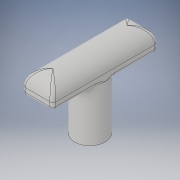
# Autodesk Inventor part: poop tray handle ver1
Saved by Autodesk Inventor 2019 (Build 230136000, 136)
## iProperties
Created: 2019-03-25
Part Number: poop tray handle ver1
Material: Generic
Document SubType Name: Modeling
Designer: aonih
Density: 1 g/cm^3
Appearance: Default
Author: aonih
Autodesk Inventor part; units mm, degrees
ref_plane "YZ Plane" through (0, 0, 0) normal (1, 0, 0) x (0, 1, 0)
ref_plane "XZ Plane" through (0, 0, 0) normal (0, 1, 0) x (-1, 0, 0)
ref_plane "XY Plane" through (0, 0, 0) normal (0, 0, 1) x (1, 0, 0)
sketch "Sketch1" plane through (0, 0, 0) normal (0, 1, 0) x (-1, 0, 0)
  circle A0 centre (0, 0) radius 5.1
  line L0 (0, 0) -> (-3.6062, -3.6062) construction
  line L1 (0, 0) -> (5.1, 0) construction
  line L2 (0, 0) -> (3.6062, 3.6062) construction
  line L3 (0, 0) -> (3.6062, -3.6062) construction
  line L4 (0, 0) -> (-3.6062, 3.6062) construction
  circle A1 centre (0, 0) radius 2.1 construction
  dimension "d7" = 135
  dimension "d8" = 5.1
  dimension "d9" = 4.2
  dimension "d10" = 3
  constraints: 10 end point, 4 point on circle, 2 centre point, 2 coincident, 1 collinear, 1 equal length, 1 horizontal, 1 perpendicular, 1 point on line
  measures "d7" angle of L0 L1
  measures "d8" distance of L0.start L0.end
  measures "d9" diameter of A1
  measures "d10" radial gap between concentric circles of A0 A1
extrude "Extrusion1" add sketch "Sketch1" along normal blind 17.5
sketch "Sketch2" plane through (0, 17.5, 0) normal (0, 1, 0) x (1, 0, 0)
  line L0 (5.1, 17.5) -> (-5.1, 17.5)
  line L1 (-5.1, 17.5) -> (-5.1, -17.5)
  line L2 (-5.1, -17.5) -> (5.1, -17.5)
  line L3 (5.1, -17.5) -> (5.1, 17.5)
  line L4 (5.1, 17.5) -> (-5.1, -17.5) construction
  line L5 (-5.1, 17.5) -> (5.1, -17.5) construction
  circle A0 centre (0, 0) radius 5.1 projected
  point P0 (-5.1, 0)
  dimension "d3" = 17.5
  dimension "d19" = 10.2
  constraints: 12 end point, 2 midpoint, 2 parallel, 1 horizontal, 1 horizontal alignment, 1 perpendicular, 1 other
  measures "d3" distance from line of point (0, 0) L2
  measures "d19" distance of L0.start L0.end
extrude "Extrusion2" add sketch "Sketch2" along normal blind 7.5
fillet "Fillet1" radius 5.1 4 edges at (5.1, 25, 0) (-5.1, 25, 0) (0, 25, 17.5) (0, 25, -17.5)
sketch "Sketch3" plane through (0, 0, 0) normal (0, -1, 0) x (1, 0, 0)
  line L0 (0, 0) -> (3.6062, -3.6062) construction
  circle A0 centre (0, 0) radius 5.1 construction
  line L1 (0, 0) -> (5.1, 0) construction
  dimension "d11" = 45
  constraints: 4 end point, 1 equal length, 1 horizontal, 2 other
  measures "d11" angle of L0 L1
hole "Hole1" at (0, 0, 0) direction (0, 1, 0) diameter 4.2 depth 8 tip angle 118
fillet "Fillet2" radius 1 4 edges at (5.1, 17.5, 8.75) (-5.1, 17.5, 8.75) (5.1, 17.5, -8.75) (-5.1, 17.5, -8.75)
fillet "Fillet3" radius 1 16 edges at (4.8071, 17.7929, 17.5) (5.1, 19.2001, 17.5) (3.6063, 23.5063, 16.0063) (0, 25, 12.4001) (-4.8071, 17.7929, 17.5) (-5.1, 19.2001, 17.5) (-3.6063, 23.5063, 16.0063) (0, 17.5, 17.5) (-4.8071, 17.7929, -17.5) (-5.1, 19.2001, -17.5) (0, 25, -12.4001) (-3.6063, 23.5063, -16.0063) (4.8071, 17.7929, -17.5) (5.1, 19.2001, -17.5) (3.6063, 23.5063, -16.0063) (0, 17.5, -17.5)
thread "Thread1" size "M5x0.8" class "6H" standard "ANSI Metric M Profile" full length
body "Solid1"
